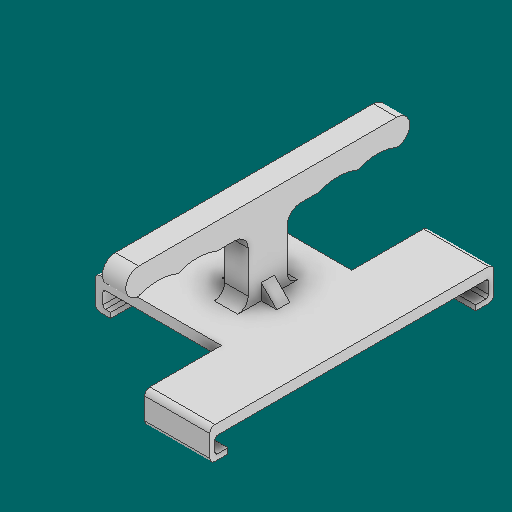
# Autodesk Inventor part: lab
Saved by Autodesk Inventor 2026.1 (Build 301233000, 233)
## iProperties
Created: 2025-10-01
Part Number: lab
Material: Genérico
Document SubType Name: Modeling
Designer: norbe
Density: 1 g/cm^3
Appearance: Valor por defecto
Author: norbe
## iProperties of the stored document lab_3DPrint.ipt
Created: 2025-10-02
Part Number: lab_3DPrint
Material: Genérico
Document SubType Name: Modeling
Designer: norbe
Density: 1 g/cm^3
Appearance: Valor por defecto
Author: norbe
Autodesk Inventor part; units mm, degrees
sketch "Boceto1" plane through (0, 0, 0) normal (0, 0, 1) x (1, 0, 0)
  line L0 (0, 0) -> (0, 6.25)
  line L1 (0, 6.25) -> (25, 6.25)
  line L2 (0, 0) -> (0, -2)
  line L3 (0, -2) -> (25, -2)
  line L4 (25, -2) -> (25, 6.25)
  line L5 (0, 0) -> (25, 0)
  line L6 (0, 10.25) -> (25, 10.25)
  line L7 (25, 10.25) -> (25, 6.25)
  line L8 (25, 6.25) -> (0, 6.25)
  line L9 (0, 6.25) -> (0, 10.25)
  dimension "d1" = 6.25
  dimension "d2" = 25
  dimension "d3" = 2
  dimension "d8" = 4
  constraints: 20 end point, 5 perpendicular, 2 parallel, 2 vertical, 1 horizontal, 1 point on line
  measures "d1" distance of L0.start L0.end
  measures "d2" distance of L0.end L1.end
  measures "d3" distance of L0.start L2.end
  measures "d8" distance of L6.end L1.end
extrude "Extrusión1" add sketch "Boceto1" against normal blind 7 contours L5 L4 L3 L2
extrude "Extrusión2" add sketch "Boceto1" against normal blind 2 contours L0 L1 L4 L5
extrude "Extrusión3" add sketch "Boceto1" against normal blind 107 contours L9 L6 L7 L1
sketch "Boceto2" plane through (0, 0, -107) normal (0, 0, -1) x (-1, 0, 0)
  line L0 (0, 0) -> (0, 6.25) projected
  line L1 (0, 6.25) -> (-25, 6.25) projected
  line L2 (-25, 6.25) -> (-25, 0) projected
  line L3 (0, 0) -> (-25, 0) projected
  line L4 (-25, -2) -> (0, -2) projected
  line L5 (-25, 0) -> (-25, -2) projected
  line L6 (-25, -2) -> (0, -2) projected
  line L7 (0, -2) -> (0, 0) projected
  line L8 (0, 0) -> (-25, 0) projected
  line L9 (0, 10.25) -> (-25, 10.25) projected
  line L10 (-25, 10.25) -> (-25, 6.25) projected
  line L11 (-25, 6.25) -> (0, 6.25) projected
  line L12 (0, 6.25) -> (0, 10.25) projected
extrude "Extrusión4" add sketch "Boceto2" along normal blind 2
extrude "Extrusión5" add sketch "Boceto2" against normal blind 5 contours L7 L4 L5 L3
ref_plane "Plano de trabajo1" through (12.5, -2, 0) normal (1, 0, 0) x (0, 0, -1)
sketch "Boceto3" plane through (12.5, -2, 0) normal (1, 0, 0) x (0, 0, -1)
  line L0 (0, 0) -> (0, 12.25) projected
  line L1 (0, 0) -> (7, 0) projected
  line L2 (7, 2) -> (7, 0) projected
  line L3 (2, 2) -> (7, 2) projected
  line L4 (2, 8.25) -> (2, 2) projected
  line L5 (2, 8.25) -> (107, 8.25) projected
  line L6 (107, 8.25) -> (107, 2) projected
  line L7 (107, 2) -> (102, 2) projected
  line L8 (102, 0) -> (102, 2) projected
  line L9 (102, 0) -> (109, 0) projected
  line L10 (109, 12.25) -> (109, 0) projected
  line L11 (0, 12.25) -> (109, 12.25) projected
  line L12 (0, 12.25) -> (47, 12.25)
  line L13 (47, 12.25) -> (47, 32.25)
  line L14 (42, 37.25) -> (5, 37.25)
  line L15 (0, 42.25) -> (0, 42.25)
  line L16 (5, 47.25) -> (104, 47.25)
  line L17 (54.5, 8.25) -> (54.5, 6.2605)
  line L18 (62, 12.25) -> (62, 32.25)
  line L19 (67, 37.25) -> (104, 37.25)
  line L20 (109, 42.25) -> (109, 42.25)
  arc A0 (47, 32.25) -> (42, 37.25) centre (42, 32.25) ccw
  arc A1 (67, 37.25) -> (62, 32.25) centre (67, 32.25) ccw
  arc A2 (0, 42.25) -> (4.4161, 37.2842) centre (5, 42.25) ccw
  arc A3 (5, 47.25) -> (0, 42.25) centre (5, 42.25) ccw
  arc A4 (109, 42.25) -> (104, 47.25) centre (104, 42.25) ccw
  arc A5 (104.5839, 37.2842) -> (109, 42.25) centre (104, 42.25) ccw
  arc A6 (20, 37.25) -> (5.3978, 37.4157) centre (12.5, 19.8086) ccw
  line L21 (20, 37.25) -> (20, 39.3903)
  arc A7 (35, 37.25) -> (20, 37.25) centre (27.5, 19.8086) ccw
  arc A8 (103.6022, 37.4157) -> (89, 37.25) centre (96.5, 19.8086) ccw
  arc A9 (89, 37.25) -> (74, 37.25) centre (81.5, 19.8086) ccw
  arc A10 (4.4161, 37.2842) -> (5.3978, 37.4157) centre (4.6496, 39.2705) ccw
  arc A11 (103.6022, 37.4157) -> (104.5839, 37.2842) centre (104.3504, 39.2705) ccw
  point P0 (0, 2)
  point P1 (47, 37.25)
  point P2 (0, 37.25)
  point P3 (0, 47.25)
  point P4 (62, 37.25)
  point P5 (109, 37.25)
  point P6 (35, 37.25)
  point P7 (62, 12.25)
  point P8 (74, 37.25)
  point P9 (0, 42.25)
  dimension "d15" = 47
  dimension "d16" = 25
  dimension "d17" = 47
  dimension "d19" = 10
  dimension "d21" = 5
  dimension "d22" = 5
  dimension "d23" = 5
  dimension "d24" = 15
  dimension "d25" = 2
  constraints: 26 point on circle, 20 end point, 16 tangent, 12 centre point, 12 point on line, 8 symmetric about line, 4 equal radius, 3 vertical, 2 horizontal, 1 midpoint, 1 perpendicular, 3 other
  measures "d15" distance of L0.end L12.end
  measures "d16" distance of L12.end point (47, 37.25)
  measures "d17" distance of point (47, 37.25) point (0, 37.25)
  measures "d19" distance of point (0, 37.25) point (0, 47.25)
  measures "d21" radius of A0
  measures "d22" radius of A1
  measures "d23" radius of A4
  measures "d24" distance of L14.end L21.start
  measures "d25" radius of A10
fillet "Empalme2" radius 2 4 edges at (12.5, 10.25, 0) (12.5, 10.25, -109) (12.5, -2, -109) (12.5, -2, 0)
fillet "Empalme3" radius 1 4 edges at (12.5, 0, -2) (12.5, 6.25, -2) (12.5, 6.25, -107) (12.5, 0, -107)
sketch "Boceto4" plane through (0, 0, 0) normal (-1, 0, 0) x (0, 0, 1)
  arc A0 (-2, -2) -> (0, 0) centre (-2, 0) ccw projected
  line L0 (0, 8.25) -> (0, 0) projected
  arc A1 (0, 8.25) -> (-2, 10.25) centre (-2, 8.25) ccw projected
  line L1 (-2, 10.25) -> (-107, 10.25) projected
  arc A2 (-107, 10.25) -> (-109, 8.25) centre (-107, 8.25) ccw projected
  line L2 (-109, 0) -> (-109, 8.25) projected
  arc A3 (-109, 0) -> (-107, -2) centre (-107, 0) ccw projected
  line L3 (-102, -2) -> (-107, -2) projected
  line L4 (-102, 0) -> (-102, -2) projected
  line L5 (-106, 0) -> (-102, 0) projected
  arc A4 (-107, 1) -> (-106, 0) centre (-106, 1) ccw projected
  line L6 (-107, 1) -> (-107, 5.25) projected
  arc A5 (-106, 6.25) -> (-107, 5.25) centre (-106, 5.25) ccw projected
  line L7 (-3, 6.25) -> (-106, 6.25) projected
  arc A6 (-2, 5.25) -> (-3, 6.25) centre (-3, 5.25) ccw projected
  line L8 (-2, 1) -> (-2, 5.25) projected
  arc A7 (-3, 0) -> (-2, 1) centre (-3, 1) ccw projected
  line L9 (-3, 0) -> (-7, 0) projected
  line L10 (-7, -2) -> (-7, 0) projected
  line L11 (-2, -2) -> (-7, -2) projected
  line L12 (-54.5, 10.25) -> (-54.5, 8.25)
  line L13 (-54.5, 10.25) -> (-79.5, 10.25)
  line L14 (-79.5, 10.25) -> (-79.5, 6.25)
  line L15 (-29.5, 10.25) -> (-29.5, 6.25)
  point P0 (0, 0)
  dimension "d31" = 25
  constraints: 8 end point, 2 point on line, 2 symmetric about line, 1 midpoint, 1 perpendicular, 1 vertical
  measures "d31" distance of L12.start L13.end
extrude "Extrusión7" add sketch "Boceto4" along normal blind 45.5 contours L15 L7 L14 L1
sketch "Boceto5" plane through (-45.5, 0, 0) normal (-1, 0, 0) x (0, 0, 1)
  line L0 (-29.5, 10.25) -> (-79.5, 10.25) projected
  line L1 (-79.5, 10.25) -> (-79.5, 6.25) projected
  line L2 (-79.5, 6.25) -> (-29.5, 6.25) projected
  line L3 (-29.5, 6.25) -> (-29.5, 10.25) projected
  line L4 (-79.5, 6.25) -> (-79.5, -2)
  line L5 (-79.5, -2) -> (-29.5, -2)
  line L6 (-29.5, -2) -> (-29.5, 6.25)
  line L7 (-79.5, 0) -> (-29.5, 0)
  point P0 (0, 0)
  point P1 (-102, -2)
  point P2 (-102, 0)
  constraints: 8 end point, 3 perpendicular, 2 point on line, 1 vertical
extrude "Extrusión8" add sketch "Boceto5" along normal blind 3
extrude "Extrusión9" add sketch "Boceto5" against normal blind 3 contours L6 L5 L4 L7
fillet "Empalme4" radius 1 2 edges at (-45.5, 6.25, -54.5) (-45.5, 0, -54.5)
fillet "Empalme5" radius 2 2 edges at (-48.5, -2, -54.5) (-48.5, 10.25, -54.5)
ref_plane "Plano de trabajo2" through (-11.75, 0, 0) normal (-1, 0, 0) x (0, 0, 1)
sketch "Boceto6" plane through (-11.75, 0, 0) normal (-1, 0, 0) x (0, 0, 1)
  line L0 (-47, 14.25) -> (-62, 14.25) projected
  line L1 (-47, 14.25) -> (-47, 30.25) projected
  arc A0 (-42, 35.25) -> (-47, 30.25) centre (-42, 30.25) ccw projected
  line L2 (-42, 35.25) -> (-35, 35.25) projected
  arc A1 (-20, 35.25) -> (-35, 35.25) centre (-27.5, 17.8086) ccw projected
  arc A2 (-5.3978, 35.4157) -> (-20, 35.25) centre (-12.5, 17.8086) ccw projected
  arc A3 (-5.3978, 35.4157) -> (-4.4161, 35.2842) centre (-4.6496, 37.2705) ccw projected
  arc A4 (-4.4161, 35.2842) -> (-5, 45.25) centre (-5, 40.25) ccw projected
  line L3 (-5, 45.25) -> (-104, 45.25) projected
  arc A5 (-104, 45.25) -> (-104.5839, 35.2842) centre (-104, 40.25) ccw projected
  arc A6 (-104.5839, 35.2842) -> (-103.6022, 35.4157) centre (-104.3504, 37.2705) ccw projected
  arc A7 (-89, 35.25) -> (-103.6022, 35.4157) centre (-96.5, 17.8086) ccw projected
  arc A8 (-74, 35.25) -> (-89, 35.25) centre (-81.5, 17.8086) ccw projected
  line L4 (-74, 35.25) -> (-67, 35.25) projected
  arc A9 (-62, 30.25) -> (-67, 35.25) centre (-67, 30.25) ccw projected
  line L5 (-62, 30.25) -> (-62, 14.25) projected
  line L6 (-62, 14.25) -> (-62, 9.2581)
  line L7 (-47, 14.25) -> (-47, 10.6824)
  line L8 (-47, 10.6824) -> (-62, 10.6824)
  line L9 (-29.5, 10.25) -> (-79.5, 10.25) projected
  line L10 (-47, 10.6824) -> (-47, 10.25)
  point P0 (0, 0)
  point P1 (-62, 10.25)
  constraints: 8 end point, 2 perpendicular, 2 point on line, 2 vertical
extrude "Extrusión10" add sketch "Boceto6" along normal mid plane 9
ref_plane "Plano de trabajo3" through (-7.25, 10.25, -54.5) normal (0, 0, -1) x (-1, 0, 0)
sketch "Boceto7" plane through (-7.25, 10.25, -54.5) normal (0, 0, -1) x (-1, 0, 0)
  line L0 (9, 20) -> (0, 20) projected
  line L1 (9, 0) -> (9, 20) projected
  line L2 (0, 0) -> (9, 0) projected
  line L3 (0, 20) -> (0, 0) projected
  line L4 (-7.25, 0) -> (39.25, 0) projected
  line L5 (9, 0) -> (9, 6)
  line L6 (9, 0) -> (15, 0)
  line L7 (0, 0) -> (-6, 0)
  line L8 (0, 0) -> (0, 6)
  line L9 (0, 6) -> (-6, 0)
  line L10 (9, 6) -> (15, 0)
  point P0 (-7.25, -10.25)
  dimension "d42" = 6
  dimension "d43" = 6
  dimension "d44" = 6
  dimension "d45" = 6
  constraints: 12 end point, 4 point on line
  measures "d42" distance of L1.start L5.end
  measures "d43" distance of L1.start L6.end
  measures "d44" distance of L2.start L7.end
  measures "d45" distance of L2.start L8.end
extrude "Extrusión11" add sketch "Boceto7" along normal mid plane 5 contours L10 L4 L1 | L3 L4 L9
fillet "Empalme6" radius 4 2 edges at (-11.75, 10.25, -47) (-11.75, 10.25, -62)
equation "\"d17\" = d15"
